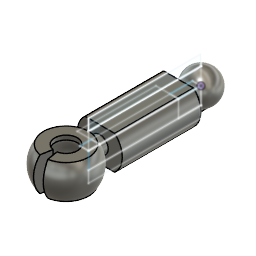
octahedron (Autodesk Fusion 360 design; units mm, degrees)
part number: 2026-08-09-08-18-06-146
Autodesk Fusion 360 part; units mm, degrees
note: some values were not read from the file. Set by a fixed rule: which sketch regions a step uses.
combine "Combine1" [no effect]
combine "Combine2" [no effect]
sketch "Sketch14" plane through (0, 0, 0) normal (0, 1, 0) x (1, 0, 0)
  circle A0 centre (0, 0) radius 1.5
  line L0 (0, 0) -> (0, 2)
  line L1 (0, 0) -> (0, -2)
  dimension "d93" = 3
  dimension "d94" = 2
  dimension "d95" = 2
  constraint coincident A0.centre L0.start
  constraint vertical L0
  constraint parallel L0 L1
  measures "d93" diameter of A0
  measures "d94" distance of A0.centre L0.end
  measures "d95" distance of A0.centre L1.end
revolve "Revolve1" add sketch "Sketch14" angle 360 about axis through (0, 0, 0) along (0, 0, 1) contours A0 L0 L1 picked at (0.7985, -0.5978) makes body 1
sketch "Sketch18" plane through (0, 0, 0) normal (0, 1, 0) x (1, 0, 0)
  line L0 (0, 0) -> (-0.75, 0)
  line L1 (-0.75, 0) -> (-0.75, -10)
  line L2 (-0.75, -10) -> (0, -10)
  line L3 (0, -10) -> (0, 0)
  line L4 (0, 0) -> (-0.75, 0)
  line L5 (-0.75, 0) -> (-0.75, -2)
  line L6 (-0.75, -2) -> (0, -2)
  line L7 (0, -2) -> (0, 0)
  line L8 (0, -10) -> (-0.75, -10)
  line L9 (-0.75, -10) -> (-0.75, -9)
  line L10 (-0.75, -9) -> (0, -9)
  line L11 (0, -9) -> (0, -10)
  line L12 (0, -9) -> (-2, -9)
  line L13 (-2, -9) -> (-2, -2)
  line L14 (-2, -2) -> (0, -2)
  line L15 (0, -2) -> (0, -9)
  dimension "d109" = 0.75
  dimension "d110" = 10
  dimension "d111" = 2
  dimension "d112" = 1
  dimension "d113" = 2
  dimension "d114" = 7
  constraint horizontal L0
  constraint vertical L1
  constraint horizontal L2
  constraint vertical L3
  constraint coincident L0.start L3.end
  constraint horizontal L4
  constraint vertical L5
  constraint horizontal L6
  constraint vertical L7
  constraint horizontal L8
  constraint vertical L9
  constraint horizontal L10
  constraint vertical L11
  constraint horizontal L12
  constraint vertical L13
  constraint horizontal L14
  constraint vertical L15
  measures "d109" distance of L0.start L0.end
  measures "d110" distance of L0.start L2.end
  measures "d111" distance of L0.start L6.end
  measures "d112" distance of L2.end L10.end
  measures "d113" distance of L10.end L12.end
  measures "d114" distance of L10.end L6.end
revolve "Revolve4" add sketch "Sketch18" angle 360 about axis through (0, 0, 10) along (0, 0, -1) separate body makes body 2
sketch "Sketch21" plane through (0, 0, 0) normal (1, 0, 0) x (0, 0, -1)
  line L0 (-10, 0) -> (-9.5, 0)
  line L1 (-9.5, 0) -> (-9.5, -0.2)
  line L2 (-9.5, -0.2) -> (-10, -0.2)
  line L3 (-10, -0.2) -> (-10, 0)
  line L4 (-9.5, -0.2) -> (-12, -0.2)
  line L5 (-12, -0.2) -> (-12, 0)
  line L6 (-12, 0) -> (-9.5, 0)
  line L7 (-9.5, 0) -> (-9.5, -0.2)
  circle A0 centre (-12, 0) radius 1.5
  circle A1 centre (-12, 0) radius 2.5
  line L8 (-9.5, 0) -> (-14.5, 0)
  line L9 (-14.5, 0) -> (-14.5, -1.5)
  line L10 (-14.5, -1.5) -> (-9.5, -1.5)
  line L11 (-9.5, -1.5) -> (-9.5, 0)
  line L12 (-14.5, -1.5) -> (-9.5, -1.5)
  line L13 (-9.5, -1.5) -> (-9.5, 1.5)
  line L14 (-9.5, 1.5) -> (-14.5, 1.5)
  line L15 (-14.5, 1.5) -> (-14.5, -1.5)
  line L16 (-12, 0) -> (-12, 3)
  line L17 (-12, 0) -> (-12, -3)
  line L18 (-12, 1.5) -> (-11, 1.5)
  line L19 (-11, 1.5) -> (-11, -1.5)
  line L20 (-11, -1.5) -> (-12, -1.5)
  line L21 (-12, -1.5) -> (-12, 1.5)
  point P0 (-10, 0)
  dimension "d129" = 0.5
  dimension "d130" = 0.2
  dimension "d131" = 2.5
  dimension "d132" = 0.2
  dimension "d133" = 3
  dimension "d134" = 5
  dimension "d135" = 5
  dimension "d136" = 1.5
  dimension "d137" = 5
  dimension "d138" = 3
  dimension "d139" = 3
  dimension "d140" = 3
  dimension "d141" = 1
  dimension "d142" = 3
  constraint horizontal L0
  constraint vertical L1
  constraint horizontal L2
  constraint vertical L3
  constraint coincident P0 L0.start
  constraint horizontal L4
  constraint vertical L5
  constraint horizontal L6
  constraint vertical L7
  constraint coincident L5.end L6.start
  constraint concentric A0 A1
  constraint horizontal L8
  constraint vertical L9
  constraint horizontal L10
  constraint vertical L11
  constraint horizontal L12
  constraint vertical L13
  constraint horizontal L14
  constraint vertical L15
  constraint perpendicular L8 L16
  constraint perpendicular L4 L17
  constraint horizontal L18
  constraint vertical L19
  constraint horizontal L20
  constraint vertical L21
  constraint midpoint L16 L18.start
  measures "d129" distance of P0 L0.end
  measures "d130" distance of P0 L2.end
  measures "d131" distance of L1.end L4.end
  measures "d132" distance of L1.end L0.end
  measures "d133" diameter of A0
  measures "d134" diameter of A1
  measures "d135" distance of L0.end L8.end
  measures "d136" distance of L0.end L10.end
  measures "d137" distance of L9.end L10.end
  measures "d138" distance of L9.end L14.end
  measures "d139" distance of L5.end L16.end
  measures "d140" distance of L5.end L17.end
  measures "d141" distance of L18.start L18.end
  measures "d142" distance of L18.start L20.end
revolve "Revolve8" add sketch "Sketch21" angle 170 about axis through (0, 0, 12) along (0, 1, 0) second angle 170 separate body contours L0 L6 A0 A1 L8 L14 L19 | L0 L2 L3 L4 L6 A1 L8 | L3 L4 L6 A0 L8 | L2 L4 A0 A1 L10 L12 L19 makes body 3
sketch "Sketch22" plane through (0, 0, 0) normal (1, 0, 0) x (0, 0, -1)
  line L0 (0, 0) -> (-10, 0)
  line L1 (-10, 0) -> (-10, 1.5)
  line L2 (-10, 1.5) -> (0, 1.5)
  line L3 (0, 1.5) -> (0, 0)
  line L4 (0, 0) -> (-10, 0)
  line L5 (-10, 0) -> (-10, -1.5)
  line L6 (-10, -1.5) -> (0, -1.5)
  line L7 (0, -1.5) -> (0, 0)
  line L8 (0, -1.5) -> (-10, -1.5)
  line L9 (-10, -1.5) -> (-10, -2.5)
  line L10 (-10, -2.5) -> (0, -2.5)
  line L11 (0, -2.5) -> (0, -1.5)
  line L12 (0, 1.5) -> (-10, 1.5)
  line L13 (-10, 1.5) -> (-10, 2.5)
  line L14 (-10, 2.5) -> (0, 2.5)
  line L15 (0, 2.5) -> (0, 1.5)
  line L16 (0, -1.5) -> (-2, -1.5)
  line L17 (-2, -1.5) -> (-2, 0)
  line L18 (-2, 0) -> (0, 0)
  line L19 (0, 0) -> (0, -1.5)
  dimension "d145" = 10
  dimension "d146" = 1.5
  dimension "d147" = 1.5
  dimension "d148" = 10
  dimension "d149" = 1
  dimension "d150" = 10
  dimension "d151" = 1
  dimension "d154" = 2
  constraint horizontal L0
  constraint vertical L1
  constraint horizontal L2
  constraint vertical L3
  constraint coincident L0.start L3.end
  constraint horizontal L4
  constraint vertical L5
  constraint horizontal L6
  constraint vertical L7
  constraint horizontal L8
  constraint vertical L9
  constraint horizontal L10
  constraint vertical L11
  constraint horizontal L12
  constraint vertical L13
  constraint horizontal L14
  constraint vertical L15
  constraint horizontal L16
  constraint vertical L17
  constraint horizontal L18
  constraint vertical L19
  measures "d145" distance of L0.start L0.end
  measures "d146" distance of L0.start L2.end
  measures "d147" distance of L0.start L6.end
  measures "d148" distance of L6.end L5.end
  measures "d149" distance of L6.end L10.end
  measures "d150" distance of L2.end L1.end
  measures "d151" distance of L2.end L14.end
  measures "d154" distance of L6.end L16.end
extrude "Extrude1" cut sketch "Sketch22" along normal mid plane 10 contours L2 L12 L13 L14 L15 | L6 L8 L9 L10 L11 L16 bodies 2
extrude "Extrude2" add sketch "Sketch22" along normal mid plane 1 separate body contours L0 L4 L6 L7 L8 L16 L17 L18 L19 makes body 4
